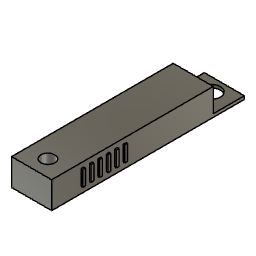
Knife blade box_ (Autodesk Fusion 360 design; units mm, degrees)
Autodesk Fusion 360 part; units mm, degrees
sketch "Sketch1" plane through (0, 0, 0) normal (0, 0, 1) x (1, 0, 0)
  line L0 (0, 0) -> (-12.9, 0)
  line L1 (-12.9, 0) -> (-12.9, 62)
  line L2 (-12.9, 62) -> (0, 62)
  line L3 (0, 62) -> (0, 0)
  circle A0 centre (-6.45, 57.75) radius 2.95
  line L4 (-12.9, 62) -> (0, 62)
  line L5 (0, 62) -> (0, 52)
  line L6 (0, 52) -> (-12.9, 52)
  line L7 (-12.9, 52) -> (-12.9, 62)
  line L8 (-12.9, 9.5) -> (-13.4, 9.5)
  line L9 (-13.4, 9.5) -> (-13.4, 10.4)
  line L10 (-13.4, 10.4) -> (-12.9, 10.4)
  line L11 (-12.9, 10.4) -> (-12.9, 9.5)
  line L12 (-12.9, 13.1) -> (-13.4, 13.1)
  line L13 (-13.4, 13.1) -> (-13.4, 12.2)
  line L14 (-13.4, 12.2) -> (-12.9, 12.2)
  line L15 (-12.9, 12.2) -> (-12.9, 13.1)
  line L16 (-12.9, 14.9) -> (-13.4, 14.9)
  line L17 (-13.4, 14.9) -> (-13.4, 15.8)
  line L18 (-13.4, 15.8) -> (-12.9, 15.8)
  line L19 (-12.9, 15.8) -> (-12.9, 14.9)
  line L20 (-12.9, 17.6) -> (-13.4, 17.6)
  line L21 (-13.4, 17.6) -> (-13.4, 18.5)
  line L22 (-13.4, 18.5) -> (-12.9, 18.5)
  line L23 (-12.9, 18.5) -> (-12.9, 17.6)
  line L24 (-12.9, 20.3) -> (-13.4, 20.3)
  line L25 (-13.4, 20.3) -> (-13.4, 21.2)
  line L26 (-13.4, 21.2) -> (-12.9, 21.2)
  line L27 (-12.9, 21.2) -> (-12.9, 20.3)
  line L28 (-12.9, 23) -> (-13.4, 23)
  line L29 (-13.4, 23) -> (-13.4, 23.9)
  line L30 (-13.4, 23.9) -> (-12.9, 23.9)
  line L31 (-12.9, 23.9) -> (-12.9, 23)
  line L32 (0.5, 23.9) -> (0, 23.9)
  line L33 (0.5, 23) -> (0.5, 23.9)
  line L34 (0, 23) -> (0.5, 23)
  line L35 (0.5, 21.2) -> (0, 21.2)
  line L36 (0.5, 20.3) -> (0.5, 21.2)
  line L37 (0, 20.3) -> (0.5, 20.3)
  line L38 (0.5, 18.5) -> (0, 18.5)
  line L39 (0.5, 17.6) -> (0.5, 18.5)
  line L40 (0, 17.6) -> (0.5, 17.6)
  line L41 (0.5, 15.8) -> (0, 15.8)
  line L42 (0.5, 14.9) -> (0.5, 15.8)
  line L43 (0, 14.9) -> (0.5, 14.9)
  line L44 (0, 13.1) -> (0.5, 13.1)
  line L45 (0.5, 13.1) -> (0.5, 12.2)
  line L46 (0.5, 12.2) -> (0, 12.2)
  line L47 (0.5, 10.4) -> (0, 10.4)
  line L48 (0.5, 9.5) -> (0.5, 10.4)
  line L49 (0, 9.5) -> (0.5, 9.5)
  circle A1 centre (-6.45, 5.25) radius 2.25
  dimension "d1" = 12.9
  dimension "d2" = 62
  dimension "d3" = 5.9
  dimension "d4" = 4.25
  dimension "d5" = 6.45
  dimension "d6" = 10
  dimension "d7" = 0.5
  dimension "d8" = 0.9
  dimension "d9" = 9.5
  dimension "d10" = 0.5
  dimension "d11" = 0.9
  dimension "d12" = 0.5
  dimension "d13" = 0.9
  dimension "d14" = 0.5
  dimension "d15" = 0.9
  dimension "d16" = 0.9
  dimension "d17" = 0.5
  dimension "d18" = 0.9
  dimension "d19" = 1.8
  dimension "d20" = 2.7
  dimension "d21" = 1.8
  dimension "d22" = 1.8
  dimension "d23" = 1.8
  dimension "d24" = 4.5
  dimension "d25" = 5.25
  dimension "d26" = 6.45
  constraint horizontal L0
  constraint vertical L1
  constraint horizontal L2
  constraint vertical L3
  constraint coincident L0.start L3.end
  constraint horizontal L4
  constraint vertical L5
  constraint horizontal L6
  constraint vertical L7
  constraint horizontal L8
  constraint vertical L9
  constraint horizontal L10
  constraint vertical L11
  constraint coincident L1 L8.start
  constraint horizontal L12
  constraint vertical L13
  constraint horizontal L14
  constraint vertical L15
  constraint coincident L1 L12.start
  constraint horizontal L16
  constraint vertical L17
  constraint horizontal L18
  constraint vertical L19
  constraint coincident L1 L16.start
  constraint horizontal L20
  constraint vertical L21
  constraint horizontal L22
  constraint vertical L23
  constraint coincident L1 L20.start
  constraint horizontal L24
  constraint vertical L25
  constraint horizontal L26
  constraint vertical L27
  constraint horizontal L28
  constraint vertical L29
  constraint horizontal L30
  constraint vertical L31
  constraint coincident L1 L28.start
  measures "d1" distance of L0.start L0.end
  measures "d2" distance of L0.start L2.end
  measures "d3" diameter of A0
  measures "d4" distance of L2 A0.centre
  measures "d5" distance of L1 A0.centre
  measures "d6" distance of L1.end L6.end
  measures "d7" distance of L8.start L8.end
  measures "d8" distance of L8.start L10.end
  measures "d9" distance of L0.end L8.start
  measures "d10" distance of L12.start L12.end
  measures "d11" distance of L12.start L14.end
  measures "d12" distance of L16.start L16.end
  measures "d13" distance of L16.start L18.end
  measures "d14" distance of L20.start L20.end
  measures "d15" distance of L20.start L22.end
  measures "d16" distance of L24.start L26.end
  measures "d17" distance of L28.start L28.end
  measures "d18" distance of L28.start L30.end
  measures "d19" distance of L10.end L14.end
  measures "d20" distance of L14.end L16.start
  measures "d21" distance of L18.end L20.start
  measures "d22" distance of L22.end L24.start
  measures "d23" distance of L26.end L28.start
  measures "d24" diameter of A1
  measures "d25" distance of L0 A1.centre
  measures "d26" distance of L3 A1.centre
extrude "Extrude1" add sketch "Sketch1" along normal blind 1 contours L1 L2 L3 L4 L5 L6 L7
extrude "Extrude2" add sketch "Sketch1" along normal blind 8.6 contours L0 L1 L3 L6 L11 L15 L19 L23 L27 L31
extrude "Extrude3" add sketch "Sketch1" along normal blind 7 contours L3 L47 L48 L49 | L1 L8 L9 L10 L11 | L3 L44 L45 L46 | L1 L12 L13 L14 L15 | L3 L41 L42 L43 | L1 L16 L17 L18 L19 | L3 L38 L39 L40 | L1 L20 L21 L22 L23 | L3 L35 L36 L37 | L1 L24 L25 L26 L27 | L3 L32 L33 L34 | L1 L28 L29 L30 L31
sketch "Sketch2" plane through (0, 0, 0) normal (0, 0, 1) x (1, 0, 0)
  line L0 (0, 0) -> (22, 0)
  line L1 (22, 0) -> (22, 28)
  line L2 (22, 28) -> (0, 28)
  line L3 (0, 28) -> (0, 0)
  line L4 (-13, 0) -> (-34, 0)
  line L5 (-34, 0) -> (-34, 25)
  line L6 (-34, 25) -> (-13, 25)
  line L7 (-13, 25) -> (-13, 0)
  constraint horizontal L0
  constraint vertical L1
  constraint horizontal L2
  constraint vertical L3
  constraint coincident L0.start L3.end
  constraint horizontal L4
  constraint vertical L5
  constraint horizontal L6
  constraint vertical L7
extrude "Extrude4" cut sketch "Sketch2" along normal blind 2
equation "d4 = d3 / 2 + 1.3 mm"
equation "d5 = d3 / 2 + ( d1 - d3 ) / 2"
equation "d20 = 1.8 mm + d13"
equation "d25 = d24 / 2 + 3 mm"
equation "d26 = d24 / 2 + ( d1 - d24 ) / 2"
